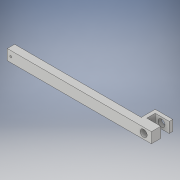
# Autodesk Inventor part: shooter launch bar
Saved by Autodesk Inventor 2019 (Build 230136000, 136)
## iProperties
Created: 2019-04-13
Part Number: shooter launch bar
Material: Generic
Document SubType Name: Modeling
Designer: Delta
Density: 1 g/cm^3
Appearance: Default
Author: Delta
Autodesk Inventor part; units mm, degrees
ref_plane "YZ Plane" through (0, 0, 0) normal (1, 0, 0) x (0, 1, 0)
ref_plane "XZ Plane" through (0, 0, 0) normal (0, 1, 0) x (-1, 0, 0)
ref_plane "XY Plane" through (0, 0, 0) normal (0, 0, 1) x (1, 0, 0)
sketch "Sketch1" plane through (0, 0, 0) normal (0, 1, 0) x (-1, 0, 0)
  line L0 (0, 0) -> (31.75, 0)
  line L1 (31.75, 0) -> (31.75, 25.4)
  line L2 (31.75, 25.4) -> (261.62, 25.4)
  line L3 (261.62, 25.4) -> (261.62, 38.735)
  line L4 (261.62, 38.735) -> (0, 38.735)
  line L5 (0, 38.735) -> (0, 0)
  line L6 (0, 21.59) -> (25.4, 21.59)
  line L7 (25.4, 21.59) -> (25.4, 6.35)
  line L8 (25.4, 6.35) -> (0, 6.35)
  line L9 (0, 6.35) -> (0, 21.59)
  dimension "d9" = 31.75
  dimension "d10" = 25.4
  dimension "d17" = 261.62
  dimension "d24" = 38.735
  dimension "d26" = 15.24
  dimension "d27" = 6.35
  dimension "d50" = 229.87
  dimension "d51" = 6.35
  constraints: 20 end point, 3 horizontal, 3 parallel, 3 perpendicular, 1 point on line
  measures "d9" distance of L0.start L0.end
  measures "d10" distance of L1.end L0.end
  measures "d17" distance of L4.end L3.end
  measures "d24" distance between parallel lines of L0 L4
  measures "d26" distance of L6.end L7.end
  measures "d27" distance between parallel lines of L0 L8
  measures "d50" distance of L1.end L2.end
  measures "d51" distance from line of L1 L7.end
extrude "Extrusion1" add sketch "Sketch1" along normal blind 19.05 contours L5 L8 L7 L6 L4 L3 L2 L1 L0
sketch "Sketch2" plane through (-261.62, 0, 38.735) normal (0, 0, 1) x (1, 0, 0)
  line L0 (261.62, 0) -> (261.62, 19.05) projected
  line L1 (0, 19.05) -> (261.62, 19.05) projected
  point P0 (247.65, 9.525)
  dimension "d37" = 13.97
  dimension "d38" = 19.05
  dimension "d39" = 9.525
  measures "d37" distance from line of L0 point (247.65, 9.525)
  measures "d38" distance of L0.start L0.end
  measures "d39" distance from line of L1 point (247.65, 9.525)
hole "Hole1" at (-13.97, 9.525, 38.735) direction (0, 0, -1) diameter 12.827 end through all
sketch "Sketch3" plane through (-261.62, 0, 38.735) normal (0, 0, 1) x (1, 0, 0)
  line L0 (0, 0) -> (0, 19.05) projected
  line L1 (0, 19.05) -> (261.62, 19.05) projected
  point P0 (261.62, 0)
  point P1 (6.35, 9.525)
  dimension "d47" = 19.05
  dimension "d48" = 9.525
  dimension "d49" = 6.35
  measures "d47" distance of L0.start L0.end
  measures "d48" distance from line of L1 point (6.35, 9.525)
  measures "d49" distance from line of L0 point (6.35, 9.525)
hole "Hole2" at (-255.27, 9.525, 38.735) direction (0, 0, -1) diameter 3.429 end through all
equation "\"d50\" = d17 - d9"
equation "\"d39\" = 0.5 * d38"
equation "\"d48\" = 0.5 * d47"
body "Solid1"
